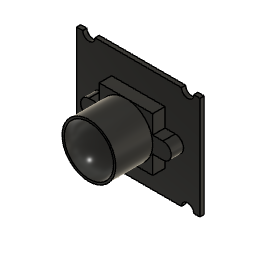
爪子 v6 (Autodesk Fusion 360 archive; units mm, degrees)
design "USB摄像头"
Autodesk Fusion 360 part; units mm, degrees
sketch "草图1" plane through (0, 0, 0) normal (0, 1, 0) x (1, 0, 0)
  line L0 (15, 12.5) -> (-15, 12.5)
  line L1 (-15, 12.5) -> (-15, -12.5)
  line L2 (-15, -12.5) -> (15, -12.5)
  line L3 (15, -12.5) -> (15, 12.5)
  line L4 (15, 12.5) -> (-15, -12.5) construction
  line L5 (-15, 12.5) -> (15, -12.5) construction
  line L6 (-18, 0) -> (20, 0)
  line L7 (0, -18) -> (0, 24)
  circle A0 centre (-12, -12.5) radius 1.5
  circle A1 centre (12, -12.5) radius 1.5
  circle A2 centre (-12, 12.5) radius 1.5
  circle A3 centre (12, 12.5) radius 1.5
  dimension "d1" = 30
  dimension "d2" = 25
  dimension "d3" = 3
  dimension "d4" = 24
  dimension "d5" = 25
  constraint horizontal L0
  constraint perpendicular L0 L1
  constraint parallel L0 L2
  constraint parallel L1 L3
  constraint coincident L4 origin
  constraint coincident L5 origin
  constraint perpendicular L3 L6
  constraint vertical L7
  constraint symmetric L7 A0 A1
  constraint symmetric L6 A0 A2
  constraint symmetric L6 A1 A3
  measures "d1" distance of L0.start L0.end
  measures "d2" distance of L0.end L1.end
  measures "d3" diameter of A0
  measures "d4" distance of A2.centre A3.centre
  measures "d5" distance of A0.centre A2.centre
extrude "拉伸1" add sketch "草图1" along normal blind 1 contours L0 L3 L6 L7 A3 | L2 L3 L6 L7 A1 | L1 L2 L6 L7 A0 | L0 L1 L6 L7 A2 makes body 1
sketch "草图2" plane through (0, 0, 0) normal (0, -1, 0) x (1, 0, 0)
  line L0 (15, 12.5) -> (13.5, 12.5)
  arc A0 (10.5, 12.5) -> (13.5, 12.5) centre (12, 12.5) ccw
  line L1 (10.5, 12.5) -> (-10.5, 12.5)
  arc A1 (-13.5, 12.5) -> (-10.5, 12.5) centre (-12, 12.5) ccw
  line L2 (-13.5, 12.5) -> (-15, 12.5)
  line L3 (-15, 12.5) -> (-15, -12.5)
  line L4 (-15, -12.5) -> (-13.5, -12.5)
  arc A2 (-10.5, -12.5) -> (-13.5, -12.5) centre (-12, -12.5) ccw
  line L5 (-10.5, -12.5) -> (10.5, -12.5)
  arc A3 (13.5, -12.5) -> (10.5, -12.5) centre (12, -12.5) ccw
  line L6 (13.5, -12.5) -> (15, -12.5)
  line L7 (15, -12.5) -> (15, 12.5)
  line L8 (6.5, -6.5) -> (-6.5, -6.5)
  line L9 (-6.5, -6.5) -> (-6.5, 6.5)
  line L10 (-6.5, 6.5) -> (6.5, 6.5)
  line L11 (6.5, 6.5) -> (6.5, -6.5)
  line L12 (6.5, -6.5) -> (-6.5, 6.5) construction
  line L13 (-6.5, -6.5) -> (6.5, 6.5) construction
  circle A4 centre (-9, 0) radius 2
  line L14 (0, 13.0883) -> (0, -18)
  circle A5 centre (9, 0) radius 2
  line L15 (-9, 2) -> (-6.5, 2)
  line L16 (-9, -2) -> (-6.5, -2)
  line L17 (9, 2) -> (6.5, 2)
  line L18 (9, -2) -> (6.5, -2)
  dimension "d8" = 13
  dimension "d9" = 13
  dimension "d10" = 4
  dimension "d11" = 18
  constraint horizontal L8
  constraint perpendicular L8 L9
  constraint parallel L8 L10
  constraint parallel L9 L11
  constraint coincident L12 origin
  constraint coincident L13 origin
  constraint perpendicular L1 L14
  constraint symmetric A4 L14 A5
  constraint coincident A4 L15.start
  constraint coincident L9 L15.end
  constraint perpendicular L9 L15
  constraint coincident A4 L16.start
  constraint coincident L9 L16.end
  constraint perpendicular L9 L16
  constraint tangent A4 L15
  constraint tangent A4 L16
  constraint coincident A5 L17.start
  constraint coincident L11 L17.end
  constraint perpendicular L11 L17
  constraint coincident A5 L18.start
  constraint coincident L11 L18.end
  constraint perpendicular L11 L18
  constraint tangent A5 L17
  constraint tangent A5 L18
  measures "d8" distance of L8.start L8.end
  measures "d9" distance of L8.end L9.end
  measures "d10" diameter of A4
  measures "d11" distance of A4.centre A5.centre
extrude "拉伸2" add sketch "草图2" along normal blind 3 separate body contours L8 L9 L10 L14 | L8 L10 L11 L14 | L9 A4 L15 L16 | L11 A5 L17 L18 | A4 | A5 makes body 2
sketch "草图3" plane through (0, -3, 0) normal (0, -1, 0) x (1, 0, 0)
  line L0 (9, 2) -> (6.5, 2)
  line L1 (6.5, 2) -> (6.5, 6.5)
  line L2 (6.5, 6.5) -> (-6.5, 6.5)
  line L3 (-6.5, 6.5) -> (-6.5, 2)
  line L4 (-6.5, 2) -> (-9, 2)
  arc A0 (-9, 2) -> (-9, -2) centre (-9, 0) ccw
  line L5 (-9, -2) -> (-6.5, -2)
  line L6 (-6.5, -2) -> (-6.5, -6.5)
  line L7 (-6.5, -6.5) -> (6.5, -6.5)
  line L8 (6.5, -6.5) -> (6.5, -2)
  line L9 (6.5, -2) -> (9, -2)
  arc A1 (9, -2) -> (9, 2) centre (9, 0) ccw
  circle A2 centre (0, 0) radius 6.5
  dimension "d14" = 13
  constraint coincident A2.centre origin
  measures "d14" diameter of A2
extrude "拉伸3" add sketch "草图3" along normal blind 9 contours A2 bodies 2
sphere "球体基本要素1" cut diameter 12 placed x (1, 0, 0) y (0, 0, 1) z (0, -1, 0) at (0, -12, 0) bodies 2
sketch "草图6" plane through (0, 1, 0) normal (0, 1, 0) x (-1, 0, 0)
  line L0 (-13.5, 12.5) -> (-15, 12.5)
  line L1 (-15, 12.5) -> (-15, -12.5)
  line L2 (-15, -12.5) -> (-13.5, -12.5)
  arc A0 (-10.5, -12.5) -> (-13.5, -12.5) centre (-12, -12.5) ccw
  line L3 (-10.5, -12.5) -> (10.5, -12.5)
  arc A1 (13.5, -12.5) -> (10.5, -12.5) centre (12, -12.5) ccw
  line L4 (13.5, -12.5) -> (15, -12.5)
  line L5 (15, -12.5) -> (15, 12.5)
  line L6 (15, 12.5) -> (13.5, 12.5)
  arc A2 (10.5, 12.5) -> (13.5, 12.5) centre (12, 12.5) ccw
  line L7 (10.5, 12.5) -> (-10.5, 12.5)
  arc A3 (-13.5, 12.5) -> (-10.5, 12.5) centre (-12, 12.5) ccw
  line L8 (-5, -8.5) -> (5, -8.5)
  line L9 (5, -8.5) -> (5, -12.5)
  line L10 (5, -12.5) -> (-5, -12.5)
  line L11 (-5, -12.5) -> (-5, -8.5)
  line L12 (0, 1) -> (0, -20)
  dimension "d18" = 10
  dimension "d19" = 4
  constraint horizontal L8
  constraint vertical L9
  constraint horizontal L10
  constraint vertical L11
  constraint coincident L3 L9.end
  constraint vertical L12
  constraint symmetric L9 L11 L12
  constraint coincident origin L12
  measures "d18" distance of L8.start L8.end
  measures "d19" distance of L8.start L10.end
extrude "拉伸4" add sketch "草图6" along normal blind 6 separate body contours L3 L8 L10 L11 L12 | L3 L8 L9 L10 L12 makes body 3

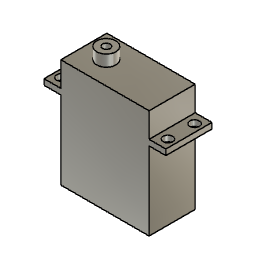
design "SCS2332舵机"
Autodesk Fusion 360 part; units mm, degrees
sketch "草图1" plane through (0, 0, 0) normal (0, 0, 1) x (1, 0, 0)
  line L0 (16, -6.05) -> (-16, -6.05)
  line L1 (-16, -6.05) -> (-16, 6.05)
  line L2 (-16, 6.05) -> (16, 6.05)
  line L3 (16, 6.05) -> (16, -6.05)
  line L4 (16, -6.05) -> (-16, 6.05) construction
  line L5 (-16, -6.05) -> (16, 6.05) construction
  line L6 (-18, 0) -> (25, 0)
  line L7 (0, 20) -> (0, -24)
  circle A0 centre (-14, 3.5) radius 1.25
  circle A1 centre (14, 3.5) radius 1.25
  circle A2 centre (-14, -3.5) radius 1.25
  circle A3 centre (14, -3.5) radius 1.25
  dimension "d1" = 12.1
  dimension "d2" = 32
  dimension "d4" = 2.5
  dimension "d5" = 28
  dimension "d6" = 7
  constraint horizontal L0
  constraint perpendicular L0 L1
  constraint parallel L0 L2
  constraint parallel L1 L3
  constraint coincident L4 origin
  constraint coincident L5 origin
  constraint perpendicular L1 L6
  constraint perpendicular L2 L7
  constraint symmetric L1 L3 L7
  constraint symmetric L0 L2 L6
  constraint symmetric L7 A0 A1
  constraint symmetric L6 A0 A2
  constraint symmetric L6 A1 A3
  measures "d1" distance of L0.end L1.end
  measures "d2" distance of L1.end L2.end
  measures "d4" diameter of A0
  measures "d5" distance of A0.centre A1.centre
  measures "d6" distance of A0.centre A2.centre
extrude "拉伸1" add sketch "草图1" along normal blind 1.5 makes body 1
sketch "草图2" plane through (0, 0, 0) normal (0, 0, -1) x (1, 0, 0)
  circle A0 centre (14, -3.5) radius 1.25
  circle A1 centre (-14, -3.5) radius 1.25
  circle A2 centre (-14, 3.5) radius 1.25
  circle A3 centre (14, 3.5) radius 1.25
  line L0 (-16, -6.05) -> (16, -6.05)
  line L1 (16, -6.05) -> (16, 6.05)
  line L2 (16, 6.05) -> (-16, 6.05)
  line L3 (-16, 6.05) -> (-16, -6.05)
  line L4 (11.6, -6.05) -> (-11.6, -6.05)
  line L5 (-11.6, -6.05) -> (-11.6, 6.05)
  line L6 (-11.6, 6.05) -> (11.6, 6.05)
  line L7 (11.6, 6.05) -> (11.6, -6.05)
  line L8 (11.6, -6.05) -> (-11.6, 6.05) construction
  line L9 (-11.6, -6.05) -> (11.6, 6.05) construction
  dimension "d9" = 23.2
  dimension "d10" = 12.1
  constraint horizontal L4
  constraint perpendicular L4 L5
  constraint parallel L4 L6
  constraint parallel L5 L7
  constraint coincident L8 origin
  constraint coincident L9 origin
  measures "d9" distance of L5.end L6.end
  measures "d10" distance of L4.start L6.end
extrude "拉伸2" add sketch "草图2" along normal blind 20.5 contours L0 L2 L4 L5 L6 L7 bodies 1
sketch "草图3" plane through (0, 0, 1.5) normal (0, 0, 1) x (-1, 0, 0)
  circle A0 centre (14, 3.5) radius 1.25
  circle A1 centre (-14, 3.5) radius 1.25
  circle A2 centre (-14, -3.5) radius 1.25
  circle A3 centre (14, -3.5) radius 1.25
  line L0 (-16, -6.05) -> (16, -6.05)
  line L1 (16, -6.05) -> (16, 6.05)
  line L2 (16, 6.05) -> (-16, 6.05)
  line L3 (-16, 6.05) -> (-16, -6.05)
  line L4 (-11.6, 6.05) -> (11.6, 6.05)
  line L5 (11.6, 6.05) -> (11.6, -6.05)
  line L6 (11.6, -6.05) -> (-11.6, -6.05)
  line L7 (-11.6, -6.05) -> (-11.6, 6.05)
  line L8 (-11.6, 6.05) -> (11.6, -6.05) construction
  line L9 (11.6, 6.05) -> (-11.6, -6.05) construction
  dimension "d13" = 23.2
  dimension "d14" = 12.1
  constraint horizontal L4
  constraint perpendicular L4 L5
  constraint parallel L4 L6
  constraint parallel L5 L7
  constraint coincident L8 origin
  constraint coincident L9 origin
  constraint coincident L2 L4.start
  measures "d13" distance of L5.end L6.end
  measures "d14" distance of L4.start L6.end
extrude "拉伸3" add sketch "草图3" along normal blind 6.5 contours L0 L2 L4 L5 L6 L7 bodies 1
sketch "草图4" plane through (0, 0, 8) normal (0, 0, 1) x (-1, 0, 0)
  line L0 (-11.6, -6.05) -> (11.6, -6.05)
  line L1 (11.6, -6.05) -> (11.6, 6.05)
  line L2 (11.6, 6.05) -> (-11.6, 6.05)
  line L3 (-11.6, 6.05) -> (-11.6, -6.05)
  line L4 (11.6, 6.05) -> (11.6, -6.05)
  line L5 (11.6, -6.05) -> (16, -6.05)
  line L6 (16, -6.05) -> (16, 6.05)
  line L7 (16, 6.05) -> (11.6, 6.05)
  circle A0 centre (14, -3.5) radius 1.25
  circle A1 centre (14, 3.5) radius 1.25
  line L8 (-11.6, -6.05) -> (-11.6, 6.05)
  line L9 (-11.6, 6.05) -> (-16, 6.05)
  line L10 (-16, 6.05) -> (-16, -6.05)
  line L11 (-16, -6.05) -> (-11.6, -6.05)
  circle A2 centre (-14, 3.5) radius 1.25
  circle A3 centre (-14, -3.5) radius 1.25
  circle A4 centre (5.7, 0) radius 2.5
  circle A5 centre (5.7, 0) radius 1
  dimension "d17" = 5
  dimension "d18" = 8.3
  dimension "d19" = 2
  constraint concentric A4 A5
  measures "d17" diameter of A4
  measures "d18" horizontal distance of A0.centre A4.centre
  measures "d19" diameter of A5
extrude "拉伸4" add sketch "草图4" along normal blind 3 separate body contours A4 makes body 2

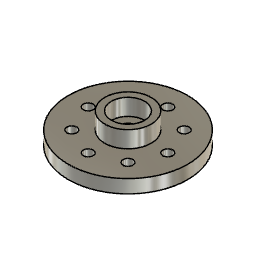
design "小舵机舵盘"
Autodesk Fusion 360 part; units mm, degrees
sketch "草图1" plane through (0, 0, 0) normal (0, 0, 1) x (1, 0, 0)
  circle A0 centre (0, 0) radius 9
  circle A1 centre (0, 0) radius 1.25
  line L0 (0, 0) -> (12.5942, 0) construction
  circle A2 centre (0, 0) radius 6 construction
  circle A3 centre (6, 0) radius 0.75
  circle A4 centre (4.2426, 4.2426) radius 0.75
  circle A5 centre (0, 6) radius 0.75
  circle A6 centre (-4.2426, 4.2426) radius 0.75
  circle A7 centre (-6, 0) radius 0.75
  circle A8 centre (-4.2426, -4.2426) radius 0.75
  circle A9 centre (0, -6) radius 0.75
  circle A10 centre (4.2426, -4.2426) radius 0.75
  dimension "d1" = 18
  dimension "d2" = 2.5
  dimension "d3" = 12
  dimension "d4" = 1.5
  dimension "d6" = 360
  constraint coincident A0.centre A1.centre
  constraint horizontal L0
  constraint concentric A0 A2
  constraint coincident A2 A3.centre
  constraint coincident L0 A3.centre
  measures "d1" diameter of A0
  measures "d2" diameter of A1
  measures "d3" diameter of A2
  measures "d4" diameter of A3
extrude "拉伸1" add sketch "草图1" along normal blind 2
sketch "草图2" plane through (0, 0, 2) normal (0, 0, 1) x (-1, 0, 0)
  circle A0 centre (6, 0) radius 0.75
  circle A1 centre (0, 6) radius 0.75
  circle A2 centre (-4.2426, -4.2426) radius 0.75
  circle A3 centre (4.2426, 4.2426) radius 0.75
  circle A4 centre (0, -6) radius 0.75
  circle A5 centre (0, 0) radius 1.25
  circle A6 centre (4.2426, -4.2426) radius 0.75
  circle A7 centre (-6, 0) radius 0.75
  circle A8 centre (-4.2426, 4.2426) radius 0.75
  circle A9 centre (0, 0) radius 9
  circle A10 centre (0, 0) radius 3.5
  circle A11 centre (0, 0) radius 2.5
  dimension "d9" = 7
  dimension "d10" = 5
  constraint concentric A5 A10
  constraint coincident A5.centre A9.centre
  measures "d9" diameter of A10
  measures "d10" diameter of A11
extrude "拉伸2" add sketch "草图2" along normal blind 2.5 contours A10
